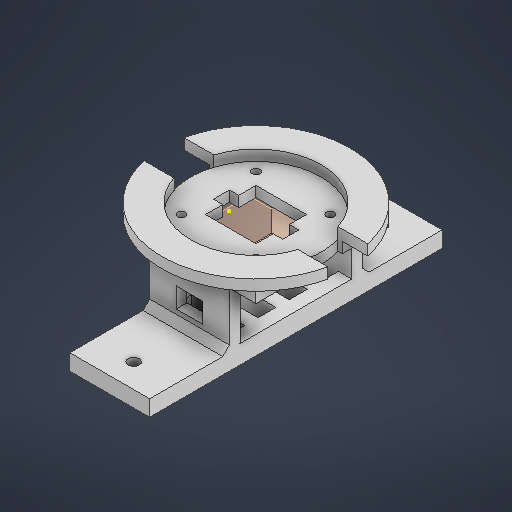
# Autodesk Inventor part: CAM1
Saved by Autodesk Inventor 2026.2 (Build 302298000, 298)
## iProperties
Created: 2025-12-02
Part Number: CAM1
Material: Generisch
Document SubType Name: Modeling
Designer: alexa
Density: 1 g/cm^3
Appearance: Vorgabe
Author: alexa
Autodesk Inventor part; units mm, degrees
ref_plane "YZ Plane" through (0, 0, 0) normal (1, 0, 0) x (0, 1, 0)
ref_plane "XZ Plane" through (0, 0, 0) normal (0, 1, 0) x (-1, 0, 0)
ref_plane "XY Plane" through (0, 0, 0) normal (0, 0, 1) x (1, 0, 0)
ref_plane "Arbeitsebene2" through (0, 0, 0) normal (0, 0, 1) x (1, 0, 0)
ref_plane "Arbeitsebene1" through (0, 0, -5) normal (0, 0, 1) x (1, 0, 0)
sketch "Skizze2" plane through (0, 0, 0) normal (0, 0, 1) x (1, 0, 0)
  line L0 (13.6, 12.5) -> (15, 12.5) projected
  arc A0 (10.4, 12.5) -> (13.6, 12.5) centre (12, 12.5) ccw projected
  line L1 (-10.4, 12.5) -> (10.4, 12.5) projected
  arc A1 (-13.6, 12.5) -> (-10.4, 12.5) centre (-12, 12.5) ccw projected
  line L2 (-15, 12.5) -> (-13.6, 12.5) projected
  line L3 (-15, 12.5) -> (-15, -12.5) projected
  line L4 (-15, -12.5) -> (-13.6, -12.5) projected
  arc A2 (-10.4, -12.5) -> (-13.6, -12.5) centre (-12, -12.5) ccw projected
  line L5 (-10.4, -12.5) -> (10.4, -12.5) projected
  arc A3 (13.6, -12.5) -> (10.4, -12.5) centre (12, -12.5) ccw projected
  line L6 (13.6, -12.5) -> (15, -12.5) projected
  line L7 (15, 12.5) -> (15, -12.5) projected
  line L8 (-8.2, 2) -> (-9, 2) projected
  arc A4 (-8.2, 2) -> (-8, 2.2) centre (-8.2, 2.2) ccw projected
  line L9 (-8, 7.8) -> (-8, 2.2) projected
  arc A5 (-7.8, 8) -> (-8, 7.8) centre (-7.8, 7.8) ccw projected
  line L10 (7.8, 8) -> (-7.8, 8) projected
  arc A6 (8, 7.8) -> (7.8, 8) centre (7.8, 7.8) ccw projected
  line L11 (8, 2.2) -> (8, 7.8) projected
  arc A7 (8, 2.2) -> (8.2, 2) centre (8.2, 2.2) ccw projected
  line L12 (9, 2) -> (8.2, 2) projected
  arc A8 (9, -2) -> (9, 2) centre (9, 0) ccw projected
  line L13 (8.2, -2) -> (9, -2) projected
  arc A9 (8.2, -2) -> (8, -2.2) centre (8.2, -2.2) ccw projected
  line L14 (8, -7.8) -> (8, -2.2) projected
  arc A10 (7.8, -8) -> (8, -7.8) centre (7.8, -7.8) ccw projected
  line L15 (-7.8, -8) -> (7.8, -8) projected
  arc A11 (-8, -7.8) -> (-7.8, -8) centre (-7.8, -7.8) ccw projected
  line L16 (-8, -2.2) -> (-8, -7.8) projected
  arc A12 (-8, -2.2) -> (-8.2, -2) centre (-8.2, -2.2) ccw projected
  line L17 (-9, -2) -> (-8.2, -2) projected
  arc A13 (-9, 2) -> (-9, -2) centre (-9, 0) ccw projected
  line L18 (-25, 25) -> (25, 25)
  line L19 (25, 25) -> (25, -25)
  line L20 (25, -25) -> (-25, -25)
  line L21 (-25, -25) -> (-25, 25)
  line L22 (0, 0) -> (0, -14)
  line L23 (0, -14) -> (14, -14)
  line L24 (14, -14) -> (14, 14)
  line L25 (14, 14) -> (-14, 14)
  line L26 (-14, 14) -> (-14, -14)
  circle A14 centre (14, -14) radius 1.5
  circle A15 centre (-14, -14) radius 1.5
  circle A16 centre (-14, 14) radius 1.5
  circle A17 centre (14, 14) radius 1.5
  dimension "d62" = 14
  dimension "d63" = 14
  dimension "d64" = 28
  dimension "d65" = 28
  dimension "d66" = 28
  dimension "d67" = 3
  dimension "d68" = 3
  dimension "d69" = 3
  dimension "d70" = 3
  constraints: 18 end point, 4 centre point, 4 coincident, 3 perpendicular, 3 vertical, 2 horizontal, 1 point on line, 4 other
  measures "d62" distance of L22.start L22.end
  measures "d63" distance of L22.end L23.end
  measures "d64" distance of L23.end L24.end
  measures "d65" distance of L24.end L25.end
  measures "d66" distance of L25.end L26.end
  measures "d67" diameter of A14
  measures "d68" diameter of A15
  measures "d69" diameter of A16
  measures "d70" diameter of A17
extrude "Extrusion1" add sketch "Skizze2" along normal blind 4 contours A0 L1 A1 L2 A16 L25 A17 L0 | L0 L24 L6 A3 L5 A2 L4 L26 L2 A1 L1 A0 | A15 | L0 L7 L6 L24 | A17 L25 L24 | L24 L25 A17 | A14 L23 L22 L5 A3 L6 | A14 L23 L24 | L24 L23 A14 | A16 L26 L25 | L25 L26 A16 | L26 L4 L3 L2 | L18 L19 L20 L21
sketch "Skizze3" plane through (0, 0, 4) normal (0, 0, 1) x (1, 0, 0)
  circle A0 centre (0, 0) radius 35.3553
  circle A1 centre (0, 0) radius 24.5
  point P0 (0, 0)
  dimension "d3" = 49
  constraints: 2 centre point, 1 coincident, 2 other
  measures "d3" diameter of A1
extrude "Extrusion2" add sketch "Skizze3" along normal blind 4
sketch "Skizze4" plane through (0, 0, 0) normal (0, 0, -1) x (-1, 0, 0)
  circle A0 centre (0, 0) radius 35.3553 projected
  line L0 (25, 25) -> (25, -25) projected
  line L1 (-25, 25) -> (25, 25)
  line L2 (25, 25) -> (25, 21)
  line L3 (25, 21) -> (-25, 21)
  line L4 (-25, 21) -> (-25, 25)
  line L5 (-25, 25) -> (0, 25)
  line L6 (-25, 25) -> (25, 25) projected
  line L7 (0, 25) -> (15, 25)
  line L8 (15, 25) -> (-15, 25)
  line L9 (-15, 25) -> (-15, 21)
  line L10 (15, 25) -> (15, 21)
  line L11 (-15, 21) -> (15, 21)
  line L12 (-35.3553, 0) -> (35.3553, 0)
  line L13 (-15, -25) -> (-15, -21)
  line L14 (15, -25) -> (15, -21)
  line L15 (-15, -21) -> (15, -21)
  line L16 (15, -25) -> (-15, -25)
  line L17 (25, -25) -> (-25, -25) projected
  line L18 (15, 25) -> (-15, 25)
  point P0 (0, 0)
  dimension "d6" = 4
  dimension "d7" = 15
  dimension "d8" = 30
  constraints: 32 end point, 5 point on line, 4 symmetric about line, 3 collinear, 3 perpendicular, 2 horizontal, 2 parallel, 1 midpoint, 4 other
  measures "d6" distance of L1.end L2.end
  measures "d7" distance of L5.end L7.end
  measures "d8" distance of L7.end L8.end
extrude "Extrusion3" add sketch "Skizze4" along normal blind 25 contours L10 L3 L9 L1 | L16 L13 L15 L14
sketch "Skizze5" plane through (-25, 25, 4) normal (0, 1, 0) x (1, 0, 0)
  line L0 (10, 29) -> (40, 29) projected
  line L1 (10, 4) -> (10, 29) projected
  line L2 (40, 29) -> (10, 29)
  line L3 (10, 29) -> (10, 25)
  line L4 (10, 25) -> (40, 25)
  line L5 (40, 25) -> (40, 29)
  line L6 (40, 29) -> (10, 29) projected
  line L7 (10, 4) -> (10, 29) projected
  point P0 (25, 4)
  dimension "d11" = 4
  constraints: 8 end point, 2 parallel, 1 horizontal, 1 perpendicular, 1 point on line
  measures "d11" distance of L3.end L2.end
sketch "Skizze6" plane through (-25, -25, 4) normal (0, -1, 0) x (1, 0, 0)
  line L0 (10, -29) -> (40, -29) projected
  line L1 (10, -4) -> (10, -29) projected
  line L2 (40, -29) -> (10, -29)
  line L3 (10, -29) -> (10, -25)
  line L4 (10, -25) -> (40, -25)
  line L5 (40, -25) -> (40, -29)
  point P0 (25, -4)
  dimension "d12" = 4
  constraints: 8 end point, 2 parallel, 1 horizontal, 1 perpendicular, 1 point on line
  measures "d12" distance of L2.end L3.end
extrude "Extrusion4" add sketch "Skizze6" along normal blind 30
extrude "Extrusion5" add sketch "Skizze5" along normal blind 30
sketch "Skizze7" plane through (-15, -21, 0) normal (0, 1, 0) x (1, 0, 0)
  line L0 (0, 25) -> (30, 25) projected
  line L1 (0, 0) -> (0, 25) projected
  line L2 (30, 0) -> (30, 25) projected
  line L3 (0, 25) -> (5, 25)
  line L4 (5, 25) -> (5, 20)
  line L5 (5, 20) -> (0, 20)
  line L6 (0, 20) -> (0, 25)
  line L7 (30, 25) -> (25, 25)
  line L8 (25, 25) -> (25, 20)
  line L9 (25, 20) -> (30, 20)
  line L10 (30, 20) -> (30, 25)
  point P0 (15, 0)
  point P1 (30, 20)
  point P2 (0, 20)
  point P3 (5, 25)
  dimension "d17" = 5
  dimension "d18" = 5
  dimension "d19" = 5
  dimension "d20" = 5
  constraints: 16 end point, 4 parallel, 2 horizontal, 2 perpendicular
  measures "d17" distance of L4.end L5.end
  measures "d18" distance of L3.end L4.end
  measures "d19" distance of L9.end L8.end
  measures "d20" distance of L8.end L7.end
extrude "Extrusion6" add sketch "Skizze7" along normal blind 44
sketch "Skizze8" plane through (0, 0, 4) normal (0, 0, 1) x (1, 0, 0)
  line L0 (-9.5, 9.5) -> (-9.5, -9.5)
  line L1 (-9.5, -9.5) -> (9.5, -9.5)
  line L2 (9.5, -9.5) -> (9.5, 9.5)
  line L3 (9.5, 9.5) -> (-9.5, 9.5)
  line L4 (-9.5, 9.5) -> (-9.5, -9.5)
  line L5 (-5, -3) -> (-5, 3)
  line L6 (-5, -3) -> (-13, -3)
  line L7 (-13, -3) -> (-13, 3)
  line L8 (-13, 3) -> (-5, 3)
  line L9 (-5, 3) -> (-5, -3)
  line L10 (5.06, -3) -> (13.06, -3)
  line L11 (13.06, -3) -> (13.06, 3)
  line L12 (13.06, 3) -> (5.06, 3)
  line L13 (5.06, 3) -> (5.06, -3)
  point P0 (0, 0)
  point P1 (-9.5, -3)
  point P2 (9.5, -3)
  point P3 (9.5, 3)
  point P4 (-9.5, 3)
  dimension "d23" = 19
  dimension "d24" = 8
  dimension "d25" = 8
  constraints: 28 end point, 6 parallel, 3 horizontal, 3 perpendicular, 2 point on line, 2 vertical, 4 other
  measures "d23" distance of L3.end L2.end
  measures "d24" distance of L7.end L8.end
  measures "d25" distance of L12.end L11.end
extrude "Extrusion7" cut sketch "Skizze8" against normal blind 15
chamfer "Fasen1" distance 2.5 angle 45 1 edges at (0, -25, -21)
chamfer "Fasen2" distance 2.5 angle 45 1 edges at (0, 25, -21)
sketch "Skizze11" plane through (-25, -25, 4) normal (0, -1, 0) x (1, 0, 0)
  line L0 (10, -4) -> (10, -22.5) projected
  line L1 (40, -22.5) -> (10, -22.5) projected
  line L2 (40, -4) -> (40, -22.5) projected
  line L3 (40, -4) -> (50, -4) projected
  line L4 (50, -4) -> (50, 0) projected
  line L5 (0, 0) -> (50, 0) projected
  line L6 (0, -4) -> (0, 0) projected
  line L7 (0, -4) -> (10, -4) projected
  line L8 (10, -4) -> (10, -22.5) projected
  line L9 (40, -22.5) -> (10, -22.5) projected
  line L10 (40, -4) -> (40, -22.5) projected
  line L11 (10, -22.5) -> (10, -25) projected
  line L12 (10, -22.5) -> (40, -22.5)
  line L13 (10, -22.5) -> (40, -22.5) projected
  line L14 (25, -22.5) -> (25, -19.5)
  line L15 (25, -19.5) -> (25, -16.5)
  line L16 (30, -19.75) -> (20, -19.75)
  line L17 (20, -19.75) -> (20, -13.25)
  line L18 (20, -13.25) -> (30, -13.25)
  line L19 (30, -13.25) -> (30, -19.75)
  line L20 (30, -19.75) -> (20, -13.25) construction
  line L21 (20, -19.75) -> (30, -13.25) construction
  point P0 (25, -4)
  point P1 (20.0696, -16.3928)
  dimension "d40" = 3
  dimension "d41" = 3
  dimension "d42" = 10
  constraints: 18 end point, 3 equal length, 3 midpoint, 2 vertical, 1 horizontal, 1 perpendicular, 1 other
  measures "d40" distance of L14.start L14.end
  measures "d41" distance of L14.end L15.end
  measures "d42" distance of L17.end L18.end
extrude "Extrusion10" cut sketch "Skizze11" against normal blind 8 contours L16 L17 L18 L19
sketch "Skizze12" plane through (-25, -25, 4) normal (0, -1, 0) x (1, 0, 0)
  line L0 (20, -13.25) -> (30, -13.25) projected
  line L1 (30, -13.25) -> (30, -19.75) projected
  line L2 (30, -19.75) -> (20, -19.75) projected
  line L3 (20, -19.75) -> (20, -13.25) projected
  line L4 (40, -22.5) -> (10, -22.5) projected
  line L5 (40, -4) -> (40, -22.5) projected
  line L6 (40, -4) -> (50, -4) projected
  line L7 (50, -4) -> (50, 0) projected
  line L8 (0, 0) -> (50, 0) projected
  line L9 (0, -4) -> (0, 0) projected
  line L10 (0, -4) -> (10, -4) projected
  line L11 (10, -4) -> (10, -22.5) projected
  line L12 (20.0696, -16.3928) -> (29.9304, -16.3928)
  line L13 (20, -19.75) -> (29.9304, -19.75)
  line L14 (29.9304, -19.75) -> (29.9304, -20.75)
  line L15 (29.9304, -20.75) -> (20, -20.75)
  line L16 (20, -20.75) -> (20, -19.75)
  point P0 (25, -4)
  dimension "d45" = 1
  constraints: 10 end point, 2 horizontal, 2 parallel, 1 perpendicular, 2 other
  measures "d45" distance of L13.end L14.end
extrude "Extrusion11" cut sketch "Skizze12" against normal blind 7.25 contours L2 L14 L15 L16
sketch "Skizze13" plane through (0, 0, 8) normal (0, 0, 1) x (1, 0, 0)
  circle A0 centre (0, 0) radius 35.3553 projected
  circle A1 centre (0, 0) radius 24.5 projected
  circle A2 centre (0, 0) radius 24.5 projected
  line L0 (-24.5, 0) -> (-36.4173, 0)
  arc A3 (-25, 25) -> (-25, -25) centre (0, 0) ccw projected
  line L1 (-35.3553, 0) -> (-35.3553, 7.5)
  line L2 (-35.3553, 7.5) -> (-23.3238, 7.5)
  line L3 (-35.3553, 0) -> (-35.3553, -7.5)
  line L4 (-35.3553, -7.5) -> (-23.3238, -7.5)
  circle A4 centre (0, 0) radius 35.3553 projected
  line L5 (0, 35.3553) -> (0, -35.3553)
  line L6 (35.3553, 0) -> (35.3553, 7.5)
  line L7 (35.3553, 7.5) -> (23.3238, 7.5)
  line L8 (35.3553, 0) -> (35.3553, -7.5)
  line L9 (35.3553, -7.5) -> (23.3238, -7.5)
  point P0 (0, 0)
  point P1 (34.5507, -7.5)
  point P2 (34.5507, 7.5)
  point P3 (-34.5507, 7.5)
  point P4 (-34.5507, -7.5)
  dimension "d48" = 7.5
  dimension "d49" = 7.5
  constraints: 20 end point, 7 point on circle, 5 symmetric about line, 3 point on line, 1 perpendicular, 1 vertical
  measures "d48" distance of L1.start L1.end
  measures "d49" distance of L1.start L3.end
extrude "Extrusion12" cut sketch "Skizze13" against normal blind 47.75 contours A0 L9 A1 L7 | L2 A1 L0 A0 | L0 A1 L4 A0
sketch "Skizze14" plane through (-10, -21, -20) normal (1, 0, 0) x (0, 0, -1)
  line L0 (0, 42) -> (5, 42) projected
  line L1 (0, 0) -> (0, 42) projected
  line L2 (5, 0) -> (0, 0) projected
  line L3 (5, 0) -> (5, 42) projected
  line L4 (5, 42) -> (5, 21)
  line L5 (5, 21) -> (0, 21)
  line L6 (0, 0) -> (0, 42) projected
  line L7 (5, 21) -> (5, 18.5)
  line L8 (5, 0) -> (5, 42) projected
  line L9 (5, 18.5) -> (0, 18.5)
  line L10 (0, 18.5) -> (0, 23.5)
  line L11 (0, 23.5) -> (5, 23.5)
  line L12 (5, 23.5) -> (5, 18.5)
  point P0 (-20, 21)
  point P1 (0, 18.5)
  point P2 (5, 18.5)
  dimension "d52" = 2.5
  dimension "d53" = 5
  constraints: 14 end point, 2 midpoint, 2 parallel, 2 point on line, 1 horizontal, 1 perpendicular
  measures "d52" distance of L4.end L7.end
  measures "d53" distance of L9.end L10.end
extrude "Extrusion13" add sketch "Skizze14" along normal blind 21.25 contours L11 L3 L5 L1 | L5 L3 L9 L1
sketch "Skizze15" plane through (-15, -55, -21) normal (0, 0, 1) x (1, 0, 0)
  line L0 (0, 27.5) -> (30, 27.5) projected
  line L1 (0, 27.5) -> (0, 0) projected
  line L2 (30, 0) -> (0, 0) projected
  line L3 (30, 27.5) -> (30, 0) projected
  line L4 (30, 82.5) -> (0, 82.5) projected
  line L5 (30, 82.5) -> (30, 110) projected
  line L6 (0, 110) -> (30, 110) projected
  line L7 (0, 82.5) -> (0, 110) projected
  line L8 (15, 0) -> (15, 9)
  circle A0 centre (15, 9) radius 2.1
  line L9 (15, 110) -> (15, 101)
  circle A1 centre (15, 101) radius 2.1
  point P0 (15, 55)
  dimension "d56" = 9
  dimension "d57" = 4.2
  dimension "d58" = 9
  dimension "d59" = 4.2
  constraints: 4 end point, 2 centre point, 2 coincident, 2 midpoint, 2 vertical
  measures "d56" distance of L8.start L8.end
  measures "d57" diameter of A0
  measures "d58" distance of L9.start L9.end
  measures "d59" diameter of A1
extrude "Extrusion14" cut sketch "Skizze15" against normal blind 41.25 contours A0 | A1
sketch "Skizze16" plane through (0, 0, 4) normal (0, 0, 1) x (1, 0, 0)
  line L0 (0, 0) -> (0, -14)
  line L1 (0, -14) -> (14, -14)
  line L2 (14, -14) -> (-14, -14)
  line L3 (-14, -14) -> (-14, 14)
  line L4 (-14, 14) -> (14, 14)
  line L5 (14, 14) -> (14, -14)
  circle A0 centre (-14, -14) radius 1.5
  circle A1 centre (-14, 14) radius 1.5
  circle A2 centre (14, 14) radius 1.5
  circle A3 centre (14, -14) radius 1.5
  dimension "d71" = 14
  dimension "d72" = 14
  dimension "d73" = 28
  dimension "d74" = 28
  dimension "d75" = 3
  dimension "d76" = 3
  dimension "d77" = 3
  dimension "d78" = 3
  constraints: 12 end point, 4 centre point, 4 coincident, 2 parallel, 2 perpendicular, 1 horizontal, 1 vertical
  measures "d71" distance of L0.start L0.end
  measures "d72" distance of L0.end L1.end
  measures "d73" distance of L3.end L4.end
  measures "d74" distance of L2.end L3.end
  measures "d75" diameter of A0
  measures "d76" diameter of A1
  measures "d77" diameter of A2
  measures "d78" diameter of A3
extrude "Extrusion15" cut sketch "Skizze16" against normal blind 7.25 contours A3 L5 L1 | L1 L5 A3 | A0 L3 L2 | L2 L3 A0 | A2 L4 L5 | L5 L4 A2 | A1 L4 L3 | L3 L4 A1
sketch "Skizze17" plane through (-10, -21, -20) normal (1, 0, 0) x (0, 0, -1)
  point P0 (-20, 21)
sketch "Skizze18" plane through (-10, -21, -20) normal (1, 0, 0) x (0, 0, -1)
  line L0 (5, 18.5) -> (0, 18.5) projected
  line L1 (0, 0) -> (0, 18.5) projected
  line L2 (5, 0) -> (0, 0) projected
  line L3 (5, 0) -> (5, 18.5) projected
  line L4 (0, 23.5) -> (5, 23.5) projected
  line L5 (5, 23.5) -> (5, 42) projected
  line L6 (0, 42) -> (5, 42) projected
  line L7 (0, 23.5) -> (0, 42) projected
  line L8 (0, 0) -> (0, 9.25)
  line L9 (0, 0) -> (0, 18.5) projected
  line L10 (0, 0) -> (0, 42) projected
  line L11 (0, 32.75) -> (0, 30.25)
  line L12 (0, 9.25) -> (0, 6.75)
  line L13 (5, 42) -> (5, -34) projected
  line L14 (0, 6.75) -> (5, 6.75)
  line L15 (5, 6.75) -> (5, 11.75)
  line L16 (5, 11.75) -> (0, 11.75)
  line L17 (0, 11.75) -> (0, 6.75)
  line L18 (0, 30.25) -> (5, 30.25)
  line L19 (5, 30.25) -> (5, 35.25)
  line L20 (5, 35.25) -> (0, 35.25)
  line L21 (0, 35.25) -> (0, 30.25)
  point P0 (-20, 21)
  point P1 (0, 35.25)
  point P2 (0, 30.25)
  point P3 (0, 6.75)
  point P4 (5, 6.75)
  dimension "d81" = 2.5
  dimension "d82" = 2.5
  dimension "d83" = 5
  dimension "d84" = 5
  constraints: 22 end point, 5 point on line, 4 parallel, 2 horizontal, 2 perpendicular, 1 midpoint
  measures "d81" distance of L11.start L11.end
  measures "d82" distance of L8.end L12.end
  measures "d83" distance of L15.end L14.end
  measures "d84" distance of L19.end L18.end
extrude "Extrusion16" add sketch "Skizze18" along normal blind 23.25 contours L3 L14 L1 L16 | L18 L7 L20 L5
sketch "Skizze19" plane through (0, 0, -25) normal (0, 0, -1) x (-1, 0, 0)
  line L0 (10, 2.5) -> (10, 9.25) projected
  line L1 (10, 2.5) -> (-10, 2.5) projected
  line L2 (-10, 2.5) -> (-10, 9.25) projected
  line L3 (10, 9.25) -> (-10, 9.25) projected
  line L4 (10, -21) -> (10, -14.25) projected
  line L5 (10, -21) -> (-10, -21) projected
  line L6 (-10, -21) -> (-10, -14.25) projected
  line L7 (10, -14.25) -> (-10, -14.25) projected
  circle A0 centre (0, 46) radius 2.1 projected
  circle A1 centre (0, -46) radius 2.1 projected
  line L8 (10, -9.25) -> (-10, -9.25) projected
  line L9 (-10, -9.25) -> (-10, -2.5) projected
  line L10 (10, -2.5) -> (-10, -2.5) projected
  line L11 (10, -9.25) -> (10, -2.5) projected
  line L12 (10, 14.25) -> (-10, 14.25) projected
  line L13 (-10, 14.25) -> (-10, 21) projected
  line L14 (-10, 21) -> (10, 21) projected
  line L15 (10, 14.25) -> (10, 21) projected
  line L16 (-15, -55) -> (-15, 55) projected
  line L17 (15, -55) -> (-15, -55) projected
  line L18 (15, 21) -> (15, -55) projected
  line L19 (15, 21) -> (15, 55) projected
  line L20 (-15, 55) -> (15, 55) projected
  point P0 (0, 0)
extrude "Extrusion17" add sketch "Skizze19" along normal blind 2
